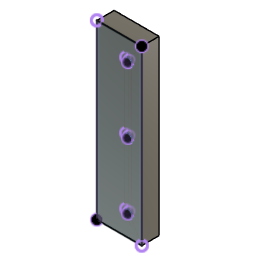
IKEA Trofast Bin to drawer bracket (Autodesk Fusion 360 design; units mm, degrees)
Autodesk Fusion 360 part; units mm, degrees
sketch "Sketch1" plane through (0, 0, 0) normal (0, 0, 1) x (1, 0, 0)
  line L0 (0, 0) -> (-26, 0)
  line L1 (-26, 0) -> (-26, -4)
  line L2 (-26, -4) -> (-13, -4)
  line L3 (-13, -4) -> (-13, -20)
  line L4 (-13, -20) -> (0, -20)
  line L5 (0, -20) -> (0, 0)
  dimension "d1" = 4
  dimension "d2" = 13
  dimension "d3" = 13
  dimension "d4" = 16
  constraint coincident L0.start L5.end
  constraint horizontal L0
  constraint perpendicular L0 L1
  constraint perpendicular L1 L2
  constraint perpendicular L0 L3
  constraint perpendicular L1 L4
  constraint perpendicular L0 L5
  measures "d1" distance of L0.end L1.end
  measures "d2" distance of L1.end L3
  measures "d3" distance of L3.end L4.end
  measures "d4" vertical distance of L1.end L3.end
extrude "Extrude1" add sketch "Sketch1" along normal blind 100 makes body 1
sketch "Sketch2" plane through (0, 0, 0) normal (0, 1, 0) x (-1, 0, 0)
  line L0 (0, 0) -> (26, 0)
  line L1 (26, 0) -> (26, 100)
  line L2 (26, 100) -> (0, 100)
  line L3 (0, 100) -> (0, 0)
  line L4 (0, 0) -> (0, 100)
  line L5 (13, 0) -> (13, 100)
  line L6 (13, 100) -> (0, 100)
  line L7 (13, 0) -> (0, 0)
  line L8 (8, 100) -> (8, 0) construction
  line L9 (8, 14.2479) -> (8, 13.9479) construction
  line L10 (9.1219, 13.9479) -> (6.8781, 13.9479)
  arc A0 (6.8781, 13.9479) -> (9.1219, 13.9479) centre (8, 12) ccw
  arc A1 (9.1219, 13.9479) -> (8, 14.2479) centre (8, 12) ccw construction
  arc A2 (8, 14.2479) -> (6.8781, 13.9479) centre (8, 12) ccw construction
  dimension "d8" = 0.3
  dimension "d10" = 12
  dimension "d11" = 4.4958
  dimension "d20" = 5
  constraint coincident L8 A0.centre
  constraint coincident L8 L9.start
  constraint coincident L8 L9.end
  constraint horizontal L10
  constraint coincident L9.end L10
  constraint concentric A0 A1
  constraint concentric A0 A2
  measures "d8" distance of L9.start L9.end
  measures "d10" distance of L8.end A0.centre
  measures "d11" diameter of A0
  measures "d20" distance of L5 L8
extrude "Extrude2" cut sketch "Sketch2" against normal through all contours L10 A0 bodies 1
pattern_linear "R-Pattern1" count 3 spacing 38 along (0, 0, 1) of "Extrude2"
fillet "Fillet1" radius 1 6 edges at (0, 0, 50) (-26, 0, 50) (-26, -4, 50) (-13, -4, 50) (-13, -20, 50) (0, -20, 50) on bodies 1
copy_body "Body->Comp1" bodies 1 removing the originals makes body 2 in component "IKEA Trofast Bin to drawer bracket"
sketch "Sketch1 (2)" plane through (0, 0, 0) normal (0, 0, 1) x (1, 0, 0) in component "Bumper"
  circle A0 centre (13.4917, 0) radius 5
  circle A1 centre (13.4917, 0) radius 2.25
  dimension "d21" = 4.5
  dimension "d22" = 10
  constraint concentric A0 A1
  measures "d21" diameter of A1
  measures "d22" diameter of A0
extrude "Extrude1'" add sketch "Sketch1 (2)" along normal blind 20 separate body makes body 3 in component "Bumper"
chamfer "Chamfer1" distance 1 angle 45 2 edges at (8.8301, -1.8081, 20) (11.394, 0.8136, 20) on bodies 3 in component "Bumper"
sketch "Sketch1 (3)" plane through (0, 0, 0) normal (0, 1, 0) x (-1, 0, 0) in component "10mm tall spacer"
  line L0 (25, 0) -> (25, 100)
  line L1 (25, 100) -> (1, 100)
  line L2 (1, 100) -> (1, 0)
  line L3 (1, 0) -> (25, 0)
  arc A0 (6.8781, 89.9479) -> (9.1219, 89.9479) centre (8, 88) ccw
  line L4 (6.8781, 89.9479) -> (9.1219, 89.9479)
  arc A1 (6.8781, 51.9479) -> (9.1219, 51.9479) centre (8, 50) ccw
  line L5 (6.8781, 51.9479) -> (9.1219, 51.9479)
  arc A2 (6.8781, 13.9479) -> (9.1219, 13.9479) centre (8, 12) ccw
  line L6 (6.8781, 13.9479) -> (9.1219, 13.9479)
  arc A3 (6.8781, 13.9479) -> (9.1219, 13.9479) centre (8, 12) ccw
  arc A4 (6.8781, 89.9479) -> (9.1219, 89.9479) centre (8, 88) ccw
  arc A5 (6.8781, 51.9479) -> (9.1219, 51.9479) centre (8, 50) ccw
  line L7 (0, 100) -> (0, 0)
  line L8 (26, 0) -> (26, 100)
  line L9 (26, 0) -> (0, 0)
  line L10 (0, 0) -> (0, 100)
  line L11 (0, 100) -> (26, 100)
  line L12 (26, 100) -> (26, 0)
  circle A6 centre (8, 12) radius 2.2479
  circle A7 centre (8, 50) radius 2.2479
  circle A8 centre (8, 88) radius 2.2479
  point P0 (26, 0)
  point P1 (0, 100)
  point P2 (26, 100)
  constraint horizontal L9
  constraint vertical L10
  constraint horizontal L11
  constraint vertical L12
  constraint coincident P1 L7.start
  constraint coincident P0 L8.start
  constraint concentric A2 A6
  constraint concentric A5 A7
  constraint concentric A4 A8
extrude "Extrude1''" add sketch "Sketch1 (3)" along normal blind 10 separate body makes body 4 in component "10mm tall spacer"
component "IKEA Trofast Bin to drawer bracket" placed x (1, 0, 0) y (0, 1, 0) z (0, 0, 1) at (0, 0, 0)
component "Bumper" placed x (1, 0, 0) y (0, 1, 0) z (0, 0, 1) at (0, 0, 0)
component "10mm tall spacer" placed x (1, 0, 0) y (0, 1, 0) z (0, 0, 1) at (0, 0, 0)
named bodies: "IKEA Trofast Bin to drawer bracket", "Bumper", "10mm tall spacer"
